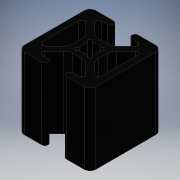
# Autodesk Inventor part: 1004-S-BLACK-FB
Saved by Autodesk Inventor 2017 SP1 (Build 210196100, 196)
## iProperties
Created: 2016-09-13
Part Number: 1004-S-BLACK-FB
Material: 6105-T5
Description: 40 S SHORT SINGLE UNIBEARING ASSEMBLY ON 40-4040 X 75mm
Document SubType Name: Modeling
Designer: BRALEF
Density: 1 g/cm^3
Appearance: BLACK ANODIZED
MATERIAL: 6061-T6
PART PRICE: 44.65
Author: BRALEF
Autodesk Inventor part; units mm, degrees
ref_plane "YZ Plane" through (0, 0, 0) normal (1, 0, 0) x (0, 1, 0)
ref_plane "XZ Plane" through (0, 0, 0) normal (0, 1, 0) x (-1, 0, 0)
ref_plane "XY Plane" through (0, 0, 0) normal (0, 0, 1) x (1, 0, 0)
sketch "Sketch1" plane through (0, 0, 0) normal (0, 1, 0) x (-1, 0, 0)
  arc A0 (-2.8605, -1.9692) -> (-1.9692, -2.8605) centre (-2.4696, -2.4696) ccw
  line L0 (-1.3405, -2.2319) -> (-1.9692, -2.8605)
  arc A1 (-1.3405, -2.2319) -> (1.3405, -2.2319) centre (0, 0) ccw
  line L1 (1.9692, -2.8605) -> (1.3405, -2.2319)
  arc A2 (1.9692, -2.8605) -> (2.8605, -1.9692) centre (2.4696, -2.4696) ccw
  line L2 (2.2319, -1.3405) -> (2.8605, -1.9692)
  arc A3 (2.2319, -1.3405) -> (2.2319, 1.3405) centre (0, 0) ccw
  line L3 (2.8605, 1.9692) -> (2.2319, 1.3405)
  arc A4 (2.8605, 1.9692) -> (1.9692, 2.8605) centre (2.4696, 2.4696) ccw
  line L4 (1.3405, 2.2319) -> (1.9692, 2.8605)
  arc A5 (1.3405, 2.2319) -> (-1.3405, 2.2319) centre (0, 0) ccw
  line L5 (-1.9692, 2.8605) -> (-1.3405, 2.2319)
  arc A6 (-1.9692, 2.8605) -> (-2.8605, 1.9692) centre (-2.4696, 2.4696) ccw
  line L6 (-2.2319, 1.3405) -> (-2.8605, 1.9692)
  arc A7 (-2.2319, 1.3405) -> (-2.2319, -1.3405) centre (0, 0) ccw
  line L7 (-2.8605, -1.9692) -> (-2.2319, -1.3405)
  arc A8 (4.5171, -1.6395) -> (5.447, -3.8845) centre (7.6921, -1.6395) ccw
  line L8 (8.7557, -7.1932) -> (5.447, -3.8845)
  arc A9 (8.7557, -7.1932) -> (10.4901, -6.4748) centre (9.4741, -6.4748) ccw
  line L9 (10.4901, 6.4748) -> (10.4901, -6.4748)
  arc A10 (10.4901, 6.4748) -> (8.7557, 7.1933) centre (9.4741, 6.4748) ccw
  line L10 (5.447, 3.8846) -> (8.7557, 7.1933)
  arc A11 (5.447, 3.8846) -> (4.5171, 1.6395) centre (7.6921, 1.6395) ccw
  line L11 (4.5171, -1.6395) -> (4.5171, 1.6395)
  arc A12 (-8.7557, 7.1933) -> (-10.4901, 6.4748) centre (-9.4741, 6.4748) ccw
  line L12 (-10.4901, -6.4747) -> (-10.4901, 6.4748)
  arc A13 (-10.4901, -6.4747) -> (-8.7557, -7.1932) centre (-9.4741, -6.4747) ccw
  line L13 (-5.4471, -3.8845) -> (-8.7557, -7.1932)
  arc A14 (-5.4471, -3.8845) -> (-4.5171, -1.6394) centre (-7.6921, -1.6394) ccw
  line L14 (-4.5171, 1.6395) -> (-4.5171, -1.6394)
  arc A15 (-4.5171, 1.6395) -> (-5.4471, 3.8846) centre (-7.6921, 1.6395) ccw
  line L15 (-8.7557, 7.1933) -> (-5.4471, 3.8846)
  arc A16 (10.5917, -12.6999) -> (12.6999, -10.5917) centre (10.5917, -10.5917) ccw
  line L16 (10.5917, -12.6999) -> (4.356, -12.6999)
  arc A17 (4.356, -10.4901) -> (4.356, -12.6999) centre (4.356, -11.595) ccw
  line L17 (4.356, -10.4901) -> (6.4748, -10.4901)
  arc A18 (6.4748, -10.4901) -> (7.1933, -8.7557) centre (6.4748, -9.4741) ccw
  line L18 (7.1933, -8.7557) -> (3.8846, -5.4471)
  arc A19 (3.8846, -5.4471) -> (1.6395, -4.5171) centre (1.6395, -7.6921) ccw
  line L19 (1.6395, -4.5171) -> (-1.6396, -4.5171)
  arc A20 (-1.6396, -4.5171) -> (-3.8847, -5.4471) centre (-1.6396, -7.6921) ccw
  line L20 (-3.8847, -5.4471) -> (-7.1933, -8.7557)
  arc A21 (-7.1933, -8.7557) -> (-6.4749, -10.4901) centre (-6.4749, -9.4741) ccw
  line L21 (-6.4749, -10.4901) -> (-4.3562, -10.4901)
  arc A22 (-4.3562, -12.6999) -> (-4.3562, -10.4901) centre (-4.3562, -11.595) ccw
  line L22 (-4.3562, -12.6999) -> (-10.5919, -12.6999)
  arc A23 (-12.7001, -10.5917) -> (-10.5919, -12.6999) centre (-10.5919, -10.5917) ccw
  line L23 (-12.7001, -10.5917) -> (-12.7001, 10.5919)
  arc A24 (-10.5919, 12.7001) -> (-12.7001, 10.5919) centre (-10.5919, 10.5919) ccw
  line L24 (-10.5919, 12.7001) -> (-4.3562, 12.7001)
  arc A25 (-4.3562, 10.4903) -> (-4.3562, 12.7001) centre (-4.3562, 11.5952) ccw
  line L25 (-4.3562, 10.4903) -> (-6.475, 10.4903)
  arc A26 (-6.475, 10.4903) -> (-7.1934, 8.7558) centre (-6.475, 9.4743) ccw
  line L26 (-7.1934, 8.7558) -> (-3.8846, 5.4471)
  arc A27 (-3.8846, 5.4471) -> (-1.6396, 4.5172) centre (-1.6396, 7.6922) ccw
  line L27 (-1.6396, 4.5172) -> (1.6395, 4.5172)
  arc A28 (1.6395, 4.5172) -> (3.8845, 5.4471) centre (1.6395, 7.6922) ccw
  line L28 (3.8845, 5.4471) -> (7.1933, 8.7558)
  arc A29 (7.1933, 8.7558) -> (6.4748, 10.4903) centre (6.4748, 9.4743) ccw
  line L29 (6.4748, 10.4903) -> (4.356, 10.4903)
  arc A30 (4.356, 12.7001) -> (4.356, 10.4903) centre (4.356, 11.5952) ccw
  line L30 (4.356, 12.7001) -> (10.5917, 12.7001)
  arc A31 (12.6999, 10.5919) -> (10.5917, 12.7001) centre (10.5917, 10.5919) ccw
  line L31 (12.6999, 10.5919) -> (12.6999, -10.5917)
  point P0 (0, 0)
  dimension "d0" = 2.1082
  dimension "d1" = 1.016
  dimension "d2" = 3.175
  dimension "d3" = 1.1049
  dimension "d4" = 0.635
  dimension "d5" = 2.6035
  dimension "d6" = 2.6035
  dimension "d7" = 2.6035
  dimension "d8" = 2.6035
  dimension "d9" = 90
  dimension "d10" = 90
  dimension "d11" = 45
  dimension "d12" = 45
  dimension "d13" = 45
  dimension "d14" = 90
  dimension "d15" = 90
  dimension "d16" = 45
  dimension "d17" = 45
  dimension "d18" = 45
  dimension "d19" = 45
  dimension "d20" = 45
  dimension "d21" = 45
  dimension "d22" = 2.2099
  dimension "d23" = 8.1829
  dimension "d24" = 17.2171
  dimension "d25" = 23.1901
  dimension "d26" = 25.4
  dimension "d27" = 1.7352
  dimension "d28" = 0.4746
  dimension "d29" = 2.2097
  dimension "d30" = 1.7351
  dimension "d31" = 0.4746
  dimension "d32" = 2.2096
  dimension "d33" = 9.0343
  dimension "d34" = 5.9731
  dimension "d35" = 15.0073
  dimension "d36" = 12.6999
  dimension "d37" = 12.7
  dimension "d38" = 12.6999
  dimension "d39" = 1.1048
  dimension "d40" = 1.1048
  dimension "d41" = 1.1049
  dimension "d42" = 1.1048
  dimension "d43" = 10.4902
  dimension "d44" = 10.4901
  dimension "d45" = 4.5172
  dimension "d46" = 0.6303
  dimension "d47" = 0.6303
  dimension "d48" = 0.6303
  dimension "d49" = 0.6303
  dimension "d50" = 1.1048
  dimension "d51" = 1.1049
  dimension "d52" = 8.3439
  dimension "d53" = 8.3439
  dimension "d54" = 9.8395
  dimension "d55" = 9.8395
  dimension "d56" = 10.2304
  dimension "d57" = 10.2304
  dimension "d58" = 10.4681
  dimension "d59" = 10.4681
  dimension "d60" = 14.6691
  dimension "d61" = 14.6691
  dimension "d62" = 15.1695
  dimension "d63" = 15.1695
  constraints: 64 end point, 64 point on circle, 48 tangent, 32 centre point, 21 equal radius, 16 parallel, 1 horizontal, 1 perpendicular, 1 vertical
  measures "d0" radius of A31
  measures "d1" radius of A10
  measures "d2" radius of A11
  measures "d3" radius of A30
  measures "d4" radius of A4
  measures "d5" radius of A7
  measures "d6" radius of A1
  measures "d7" radius of A5
  measures "d8" radius of A3
  measures "d9" angle of L30 L31
  measures "d10" angle of L31 L16
  measures "d11" angle of L31 L10
  measures "d12" angle of L31 L8
  measures "d13" angle of L31 L28
  measures "d14" angle of L31 L29
  measures "d15" angle of L31 L17
  measures "d16" angle of L31 L5
  measures "d17" angle of L31 L0
  measures "d18" angle of L31 L6
  measures "d19" angle of L31 L7
  measures "d20" angle of L31 L15
  measures "d21" angle of L31 L13
  measures "d22" distance between parallel lines of L31 L9
  measures "d23" distance between parallel lines of L31 L11
  measures "d24" distance between parallel lines of L31 L14
  measures "d25" distance between parallel lines of L31 L12
  measures "d26" distance between parallel lines of L23 L31
  measures "d27" distance between parallel lines of L3 L28
  measures "d28" distance between parallel lines of L4 L28
  measures "d29" distance between parallel lines of L20 L28
  measures "d30" distance between parallel lines of L2 L18
  measures "d31" distance between parallel lines of L1 L18
  measures "d32" distance between parallel lines of L26 L18
  measures "d33" distance between parallel lines of L27 L19
  measures "d34" distance between parallel lines of L25 L27
  measures "d35" distance between parallel lines of L27 L21
  measures "d36" distance from line of point (0, 0) L31
  measures "d37" distance from line of point (0, 0) L30
  measures "d38" distance from line of point (0, 0) L16
  measures "d39" distance from line of point (0, 0) L10
  measures "d40" distance from line of point (0, 0) L8
  measures "d41" distance from line of point (0, 0) L28
  measures "d42" distance from line of point (0, 0) L18
  measures "d43" distance from line of point (0, 0) L29
  measures "d44" distance from line of point (0, 0) L17
  measures "d45" distance from line of point (0, 0) L27
  measures "d46" distance from line of point (0, 0) L5
  measures "d47" distance from line of point (0, 0) L0
  measures "d48" distance from line of point (0, 0) L6
  measures "d49" distance from line of point (0, 0) L7
  measures "d50" distance from line of point (0, 0) L15
  measures "d51" distance from line of point (0, 0) L13
  measures "d52" distance from line of L30.start L31
  measures "d53" distance from line of L17.start L31
  measures "d54" distance from line of L3.start L31
  measures "d55" distance from line of L2.end L31
  measures "d56" distance from line of A4.centre L31
  measures "d57" distance from line of A2.centre L31
  measures "d58" distance from line of L3.end L31
  measures "d59" distance from line of L2.start L31
  measures "d60" distance from line of L5.start L31
  measures "d61" distance from line of L0.end L31
  measures "d62" distance from line of A6.centre L31
  measures "d63" distance from line of A0.centre L31
extrude "Extrusion1" add sketch "Sketch1" along normal mid plane 25.4
body "Solid1"
